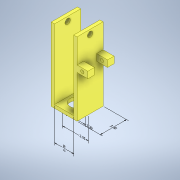
# Autodesk Inventor part: forkV02
Saved by Autodesk Inventor 2021.1 (Build 251245010, 245A)
## iProperties
Created: 2020-07-21
Part Number: forkV02
Material: PC/ABS Plastic
Document SubType Name: Modeling
Designer: robst
Density: 0.357273 g/cm^3
Appearance: Smooth - Yellow
Mass: 137.886 g
Surface Area: 962.27 cm^2
Volume: 385.941 cm^3
Author: robst
Autodesk Inventor part; units mm, degrees
ref_plane "YZ Plane" through (0, 0, 0) normal (1, 0, 0) x (0, 1, 0)
ref_plane "XZ Plane" through (0, 0, 0) normal (0, 1, 0) x (-1, 0, 0)
ref_plane "XY Plane" through (0, 0, 0) normal (0, 0, 1) x (1, 0, 0)
sketch "Sketch1" plane through (0, 0, 0) normal (0, 0, 1) x (1, 0, 0)
  line L0 (0, 0) -> (27.94, 0)
  line L1 (27.94, 0) -> (27.94, 203.2)
  line L2 (0, 0) -> (-27.94, 0)
  line L3 (-27.94, 0) -> (-27.94, 203.2)
  line L4 (-27.94, 203.2) -> (-37.465, 203.2)
  line L5 (-37.465, 203.2) -> (-37.465, -9.525)
  line L6 (-37.465, -9.525) -> (37.465, -9.525)
  line L7 (37.465, -9.525) -> (37.465, 203.2)
  line L8 (37.465, 203.2) -> (27.94, 203.2)
  dimension "d0" = 203.2
  dimension "d1" = 27.94
  dimension "x2" = 9.525
  dimension "d3" = 9.525
  dimension "d4" = 9.525
  constraints: 18 end point, 5 perpendicular, 3 horizontal, 2 equal length, 1 point on line, 1 vertical
  measures "d0" distance of L0.end L1.end
  measures "d1" distance from line of L1 L0.start
  measures "x2" distance between parallel lines of L5 L3
  measures "d3" distance between parallel lines of L2 L6
  measures "d4" distance of L7.end L1.end
extrude "Extrusion1" add sketch "Sketch1" against normal mid plane 76.2
sketch "Sketch2" plane through (37.465, -9.525, -38.1) normal (1, 0, 0) x (0, 0, -1)
  circle A0 centre (-38.1, 200.025) radius 7.9375
  point P0 (-38.1, 9.525)
  dimension "d7" = 15.875
  dimension "d8" = 190.5
  constraints: 1 centre point
  measures "d7" diameter of A0
  measures "d8" distance of A0.centre point (-38.1, 9.525)
extrude "Extrusion2" cut sketch "Sketch2" against normal through all
sketch "Sketch3" plane through (0, 0, 38.1) normal (0, 0, 1) x (1, 0, 0)
  line L0 (37.465, 203.2) -> (37.465, -9.525) projected
  line L1 (37.465, 132.461) -> (69.215, 132.461)
  line L2 (69.215, 132.461) -> (69.215, 113.411)
  line L3 (69.215, 113.411) -> (37.465, 113.411)
  line L4 (37.465, 113.411) -> (37.465, 132.461)
  line L5 (37.465, 122.936) -> (69.215, 122.936) construction
  line L6 (-37.465, -9.525) -> (37.465, -9.525) construction
  circle A0 centre (53.1368, 122.936) radius 4.7625
  point P0 (0, 0)
  point P1 (37.465, 113.411)
  dimension "d20" = 31.75
  dimension "d21" = 19.05
  dimension "d22" = 132.461
  dimension "d23" = 9.525
  dimension "d24" = 15.6718
  constraints: 10 end point, 2 midpoint, 2 parallel, 2 point on line, 1 centre point, 1 horizontal, 1 perpendicular
  measures "d20" distance of L2.end L3.end
  measures "d21" distance of L1.end L2.end
  measures "d22" distance between parallel lines of L5 L6
  measures "d23" diameter of A0
  measures "d24" distance from line of A0.centre L0
extrude "Extrusion3" add sketch "Sketch3" against normal blind 19.05
mirror "Mirror1" about plane through (0, 0, 0) normal (0, 0, 1) of "Extrusion3"
sketch "Sketch4" plane through (-37.465, -9.525, -38.1) normal (0, -1, 0) x (1, 0, 0)
  circle A0 centre (37.465, 38.1) radius 20.6375
  dimension "d27" = 41.275
  constraints: 1 centre point, 1 coincident
  measures "d27" diameter of A0
extrude "Extrusion4" cut sketch "Sketch4" against normal through all
equation "\"d0\" = overallHeight"
equation "\"x2\" = wallThickness"
equation "\"d3\" = wallThickness"
equation "\"d4\" = wallThickness"
equation "\"d5\" = overallWidth"
equation "\"d7\" = postHoleDiameter"
equation "\"d8\" = postHoleFromTop"
equation "\"postHoleDiameter\" = 15.875"
equation "\"overallHeight\" = 203.2"
equation "\"wallThickness\" = 9.525"
equation "\"overallWidth\" = 76.2"
equation "\"postHoleFromTop\" = 190.5"
body "Solid1"
